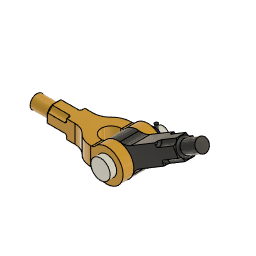
Knuckle Joint v1 (Autodesk Fusion 360 design; units mm, degrees)
Autodesk Fusion 360 part; units mm, degrees
sketch "Sketch1" plane through (0, 0, 0) normal (0, 0, 1) x (1, 0, 0) in component "Fork"
  line L0 (101.25, -47.5) -> (25.75, -47.5)
  line L1 (-101.25, -21) -> (-101.25, 21)
  line L2 (25.75, 47.5) -> (101.25, 47.5)
  line L3 (25.75, 22.5) -> (101.25, 22.5)
  line L4 (101.25, -22.5) -> (25.75, -22.5)
  line L5 (-16.8558, -21) -> (-101.25, -21)
  line L6 (-101.25, 21) -> (-16.8558, 21)
  line L7 (-101.25, 17.2472) -> (-110, 21) construction
  line L8 (0, 0) -> (3.3034, 1.5498) construction
  line L9 (3.3034, -1.5498) -> (0, 0) construction
  arc A0 (25.75, 22.5) -> (25.75, -22.5) centre (25.75, 0) ccw
  line L10 (101.25, 47.5) -> (101.25, 22.5)
  line L11 (101.25, -22.5) -> (101.25, -47.5)
  arc A1 (25.75, 47.5) -> (25.75, -47.5) centre (25.75, 0) ccw
  dimension "d3" = 45
  dimension "d4" = 95
  dimension "d5" = 75.5
  dimension "d6" = 45
  constraint horizontal L0
  constraint perpendicular L0 L1
  constraint parallel L0 L2
  constraint parallel L1 L10
  constraint coincident L8.start L9.end
  constraint concentric A0 A1
  constraint horizontal L3
  constraint horizontal L4
  constraint horizontal L5
  constraint parallel L5 L6
  constraint coincident L1 L7.start
  constraint coincident L9.end L8
  constraint coincident L8.end A0
  constraint coincident L9.start A0
  constraint collinear L10 L11
  constraint coincident A1 L5.start
  constraint coincident A1 L6.end
  measures "d3" diameter of A0
  measures "d4" diameter of A1
  measures "d5" distance of A0.centre L10
  measures "d6" distance of L3.start L4.end
extrude "Extrude1" add sketch "Sketch1" along normal mid plane 80 makes body 1 in component "Fork"
sketch "Sketch2" plane through (0, -47.5, 0) normal (0, -1, 0) x (1, 0, 0) in component "Fork"
  line L0 (101.25, -40) -> (101.25, 40)
  line L1 (101.25, 40) -> (25.75, 40)
  line L2 (25.75, 40) -> (25.75, -40)
  line L3 (25.75, -40) -> (101.25, -40)
  circle A0 centre (63.75, 0) radius 15
  circle A1 centre (63.75, 0) radius 37.5
  line L4 (32.6815, 21) -> (-116.805, 21)
  line L5 (-116.805, 21) -> (-116.805, -21)
  line L6 (-116.805, -21) -> (32.6815, -21)
  line L7 (32.6815, -21) -> (32.6815, 21)
  dimension "d10" = 30
  dimension "d11" = 75
  dimension "d12" = 42
  constraint concentric A0 A1
  constraint tangent L0 A1
  constraint horizontal L4
  constraint vertical L5
  constraint horizontal L6
  constraint vertical L7
  constraint coincident A1 L4.start
  constraint coincident A1 L6.end
  measures "d10" diameter of A0
  measures "d11" diameter of A1
  measures "d12" distance of L4.start L6.end
extrude "Extrude2" cut sketch "Sketch2" against normal blind 95 contours A1 L7 | A1 L7 | L2 A1 L4 L6 | L2 L4 L5 L6 keep common part bodies 1 in component "Fork"
fillet "Fillet1" radius 10 4 edges at (32.6815, -35, 21) (32.6815, 35, 21) (32.6815, -35, -21) (32.6815, 35, -21) on bodies 1 in component "Fork"
fillet "Fillet2" radius 40 2 edges at (-16.8558, -21, 0) (-16.8558, 21, 0) on bodies 1 in component "Fork"
sketch "Sketch3" plane through (-101.25, 0, 0) normal (-1, 0, 0) x (0, -1, 0) in component "Fork"
  line L0 (-21, -21) -> (21, -21)
  line L1 (21, -21) -> (21, 21)
  line L2 (21, 21) -> (-21, 21)
  line L3 (-21, 21) -> (-21, -21)
  circle A0 centre (21, 21) radius 10.5
  circle A1 centre (-21, 21) radius 10.5
  circle A2 centre (-21, -21) radius 10.5
  circle A3 centre (21, -21) radius 10.5
  dimension "d19" = 21
  dimension "d21" = 360
  constraint coincident L1.end L2.start
  measures "d19" diameter of A0
extrude "Extrude3" cut sketch "Sketch3" against normal blind 45 contours L0 L3 A2 | L0 L1 A3 | L2 L3 A1 | L1 L2 A0 picked at (-19.5158, -14.1774) picked at (16.8157, -15.4105) picked at (-14.0356, 20.5019) picked at (14.0356, 20.5019) bodies 1 in component "Fork"
fillet "Fillet3" radius 5 4 edges at (-56.25, -13.5754, 13.5754) (-56.25, -13.5754, -13.5754) (-56.25, 13.5754, 13.5754) (-56.25, 13.5754, -13.5754) on bodies 1 in component "Fork"
cylinder "CylinderPrimitive1" add diameter 32 height 45 placed x (0, 0, 1) y (0, 1, 0) z (-1, 0, 0) at (-101.25, 0, 0) bodies 1 in component "Fork"
fillet "Fillet4" radius 5 1 edges at (-101.25, 5.7858, -14.9172) on bodies 1 in component "Fork"
sketch "Sketch1 (2)" plane through (0, 0, 0) normal (0, 0, 1) x (1, 0, 0) in component "Eye rod"
  line L0 (-146.25, 16) -> (-146.25, -16)
  line L1 (-61.25, 21) -> (-56.25, 21)
  line L2 (-56.25, -21) -> (-61.25, -21)
  line L3 (-61.25, 21) -> (-101.25, 21)
  line L4 (-101.25, -21) -> (-61.25, -21)
  line L5 (-56.25, 21) -> (-36.9816, 21)
  arc A0 (-36.9816, 21) -> (-8.3043, 33.1143) centre (-36.9816, 61) ccw
  arc A1 (25.75, 47.5) -> (-8.3043, 33.1143) centre (25.75, 0) ccw
  line L6 (25.75, 47.5) -> (27.7604, 47.5)
  line L7 (27.7604, 22.5) -> (25.75, 22.5)
  arc A2 (25.75, 22.5) -> (25.75, -22.5) centre (25.75, 0) ccw
  line L8 (25.75, -22.5) -> (27.7604, -22.5)
  line L9 (27.7604, -47.5) -> (25.75, -47.5)
  arc A3 (-8.3043, -33.1143) -> (25.75, -47.5) centre (25.75, 0) ccw
  arc A4 (-8.3043, -33.1143) -> (-36.9816, -21) centre (-36.9816, -61) ccw
  line L10 (-36.9816, -21) -> (-56.25, -21)
  line L11 (35.3372, 22.5) -> (27.7604, 22.5)
  line L12 (27.7604, 47.5) -> (35.3372, 47.5)
  line L13 (27.7604, -22.5) -> (35.3372, -22.5)
  line L14 (35.3372, -47.5) -> (27.7604, -47.5)
  line L15 (35.3372, -22.5) -> (101.25, -22.5)
  line L16 (101.25, -47.5) -> (35.3372, -47.5)
  line L17 (35.3372, 47.5) -> (101.25, 47.5)
  line L18 (101.25, 22.5) -> (35.3372, 22.5)
  arc A5 (-106.25, 16) -> (-101.25, 21) centre (-106.25, 21) ccw
  arc A6 (-101.25, -21) -> (-106.25, -16) centre (-106.25, -21) ccw
  line L19 (-106.25, 16) -> (-146.25, 16)
  line L20 (-106.25, -16) -> (-146.25, -16)
  line L21 (101.25, -47.5) -> (101.25, -22.5)
  line L22 (101.25, 22.5) -> (101.25, 47.5)
  line L23 (26.25, 22.5) -> (221.25, 22.5)
  line L24 (221.25, 22.5) -> (221.25, -22.5)
  line L25 (221.25, -22.5) -> (26.25, -22.5)
  line L26 (26.25, -22.5) -> (26.25, 22.5)
  dimension "d30" = 45
  dimension "d31" = 75
  dimension "d32" = 195
  constraint horizontal L23
  constraint vertical L24
  constraint horizontal L25
  constraint vertical L26
  constraint coincident L18 L23.start
  measures "d30" distance of L23.start L25.end
  measures "d31" distance of L22 L26
  measures "d32" distance of L24 L26
extrude "Extrude1'" add sketch "Sketch1 (2)" along normal mid plane 80 separate body contours L7 L8 L11 L13 L15 L18 L23 L24 L25 L26 makes body 2 in component "Eye rod"
sketch "Sketch2 (2)" plane through (0, -22.5, 0) normal (0, -1, 0) x (1, 0, 0) in component "Eye rod"
  line L0 (221.25, -40) -> (221.25, 40)
  line L1 (221.25, 40) -> (26.25, 40)
  line L2 (26.25, 40) -> (26.25, -40)
  line L3 (26.25, -40) -> (221.25, -40)
  circle A0 centre (63.75, 0) radius 37.5
  circle A1 centre (63.75, 0) radius 15
  line L4 (94.8185, 21) -> (226.5764, 21)
  line L5 (226.5764, 21) -> (226.5764, -21)
  line L6 (226.5764, -21) -> (94.8185, -21)
  line L7 (94.8185, -21) -> (94.8185, 21)
  dimension "d35" = 75
  dimension "d36" = 30
  dimension "d37" = 42
  dimension "d38" = 21
  constraint concentric A0 A1
  constraint horizontal L4
  constraint vertical L5
  constraint horizontal L6
  constraint vertical L7
  constraint coincident A0 L4.start
  constraint coincident A0 L6.end
  measures "d35" diameter of A0
  measures "d36" diameter of A1
  measures "d37" distance of L4.start L6.end
  measures "d38" distance of A0.centre L4
extrude "Extrude2'" cut sketch "Sketch2 (2)" against normal blind 45 contours L0 A0 L4 L6 | A0 L7 | A0 L7 keep common part bodies 2 in component "Eye rod"
fillet "Fillet1'" radius 40 2 edges at (94.8185, 0, 21) (94.8185, 0, -21) on bodies 2 in component "Eye rod"
sketch "Sketch3 (2)" plane through (221.25, 0, 0) normal (1, 0, 0) x (0, 1, 0) in component "Eye rod"
  line L0 (22.5, 21) -> (-22.5, 21)
  line L1 (-22.5, 21) -> (-22.5, -21)
  line L2 (-22.5, -21) -> (22.5, -21)
  line L3 (22.5, -21) -> (22.5, 21)
  circle A0 centre (22.5, 21) radius 10.5
  circle A1 centre (-21, 22.5) radius 10.5
  circle A2 centre (-22.5, -21) radius 10.5
  circle A3 centre (21, -22.5) radius 10.5
  dimension "d43" = 21
  dimension "d45" = 360
  constraint coincident L0.start L3.end
  measures "d43" diameter of A0
extrude "Extrude3'" cut sketch "Sketch3 (2)" against normal blind 45 contours L0 L3 A0 | L0 L1 A1 | L2 L3 A3 | L1 L2 A2 picked at (15.5356, 20.5019) picked at (-14.6782, 20.5121) picked at (14.6782, -20.5121) picked at (-20.06, -14.4581) bodies 2 in component "Eye rod"
cylinder "CylinderPrimitive1'" add diameter 30 height 45 placed x (0, 0, -1) y (0, 1, 0) z (1, 0, 0) at (221.25, 0, 0) bodies 2 in component "Eye rod"
fillet "Fillet2'" radius 5 1 edges at (221.25, 5.4242, 13.9849) on bodies 2 in component "Eye rod"
fillet "Fillet3'" radius 5 4 edges at (176.25, -14.7122, 14.0909) (176.25, 15.0754, 13.5754) (176.25, -15.0754, -13.5754) (176.25, 14.7122, -14.0909) on bodies 2 in component "Eye rod"
sketch "Sketch1 (3)" plane through (0, -47.5, 0) normal (0, -1, 0) x (1, 0, 0) in component "Pin"
  arc A0 (35.3372, -24.4737) -> (27.7604, -21) centre (27.7604, -31) ccw
  arc A1 (35.3372, -24.4737) -> (35.3372, 24.4737) centre (63.75, 0) ccw
  arc A2 (27.7604, 21) -> (35.3372, 24.4737) centre (27.7604, 31) ccw
  line L0 (27.7604, 21) -> (25.75, 21)
  line L1 (25.75, 21) -> (25.75, -21)
  line L2 (25.75, -21) -> (27.7604, -21)
  circle A3 centre (63.75, 0) radius 15
  circle A4 centre (63.75, 0) radius 15
  circle A5 centre (63.75, 0) radius 22.5
  dimension "d54" = 30
  dimension "d55" = 45
  constraint concentric A1 A4
  constraint concentric A4 A5
  measures "d54" diameter of A4
  measures "d55" diameter of A5
extrude "Extrude1''" add sketch "Sketch1 (3)" against normal blind 130 separate body contours A3 A4 makes body 3 in component "Pin"
extrude "Extrude2''" add sketch "Sketch1 (3)" along normal blind 15 contours A3 A4 | A5 bodies 3 in component "Pin"
hole "Hole1" at (63.75, 67.5, 15) direction (0, 0, -1) diameter 7 end through all bodies 3 in component "Pin"
sketch "Sketch1 (4)" plane through (0, 47.5, 0) normal (0, 1, 0) x (-1, 0, 0) in component "Washer"
  circle A0 centre (-63.75, 0) radius 15
  line L0 (-27.7604, -21) -> (-25.75, -21)
  line L1 (-25.75, -21) -> (-25.75, 21)
  line L2 (-25.75, 21) -> (-27.7604, 21)
  arc A1 (-35.3372, 24.4737) -> (-27.7604, 21) centre (-27.7604, 31) ccw
  arc A2 (-35.3372, 24.4737) -> (-35.3372, -24.4737) centre (-63.75, 0) ccw
  arc A3 (-27.7604, -21) -> (-35.3372, -24.4737) centre (-27.7604, -31) ccw
  circle A4 centre (-63.75, 0) radius 22.5
  dimension "d63" = 45
  constraint concentric A0 A4
  measures "d63" diameter of A4
extrude "Extrude1'''" add sketch "Sketch1 (4)" along normal blind 15 separate body contours A4 makes body 4 in component "Washer"
sketch "Sketch1 (5)" plane through (0, 0, 0) normal (0, 0, 1) x (1, 0, 0)
  circle A0 through (69, 100, 45) (63, 103.4641, 45) (63, 96.5359, 45)
  circle A1 centre (65, 100) radius 3
  dimension "d67" = 8
  dimension "d68" = 6
  measures "d68" diameter of A1
loft "Loft1" add profiles "Sketch1 (5)", "Sketch1 (5)" section 1 contours A0 in plane through (0, 0, 45) normal (0, 0, 1) section 2 separate body makes body 5
copy_body "Body->Comp1" bodies 5 removing the originals makes body 6 in component "Taper Pin"
component "Eye rod" placed x (1, 0, 0) y (0, 1, 0) z (0, 0, 1) at (0, 0, 0)
component "Pin" placed x (1, 0, 0) y (0, 1, 0) z (0, 0, 1) at (0, 0, 0)
component "Washer" placed x (1, 0, 0) y (0, 1, 0) z (0, 0, 1) at (0, 0, 0)
component "Taper Pin" placed x (0.978148, 0.207912, 0) y (-0.207912, 0.978148, 0) z (0, 0, 1) at (20.9616, -43.829, -17.998)
component "Fork" placed x (1, 0, 0) y (0, 1, 0) z (0, 0, 1) at (0, 0, 0)
